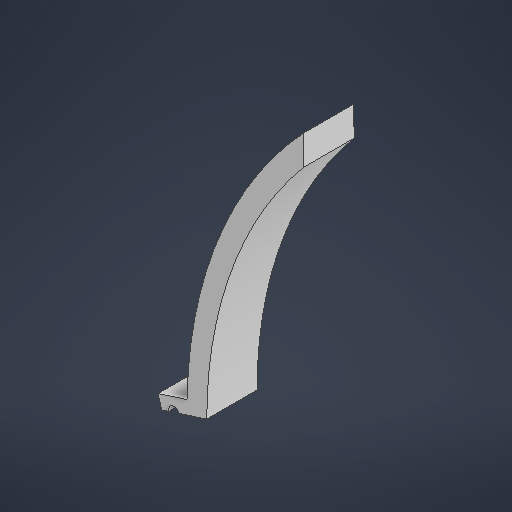
# Autodesk Inventor part: направление
Saved by Autodesk Inventor 2025 (Build 290162000, 162)
## iProperties
Created: 2025-11-04
Part Number: направление
Material: Типовые
Document SubType Name: Modeling
Designer: GameHD
Density: 1 g/cm^3
Appearance: По умолчанию
Author: GameHD
Autodesk Inventor part; units mm, degrees
ref_plane "YZ Plane" through (0, 0, 0) normal (1, 0, 0) x (0, 1, 0)
ref_plane "XZ Plane" through (0, 0, 0) normal (0, 1, 0) x (-1, 0, 0)
ref_plane "XY Plane" through (0, 0, 0) normal (0, 0, 1) x (1, 0, 0)
sketch "Эскиз1" plane through (0, 0, 0) normal (0, 0, 1) x (1, 0, 0)
  circle A0 centre (0, 0) radius 165
  circle A1 centre (0, 0) radius 172.834
  line L0 (-125, 0) -> (-126.5392, 117.7261)
  line L1 (-132.7592, 119.5177) -> (-197.8467, 76.6552)
  line L2 (-165, 0) -> (-153, 0) construction
  line L3 (-134.7038, 9.8338) -> (-172.765, -2.5204) projected
  line L4 (-165, 0) -> (-172.8154, -2.5368)
  point P0 (-172.834, 0)
  point P1 (-126.3868, 106.0725)
  point P2 (-123, 114.4334)
  point P3 (-172.8149, -2.5694)
  dimension "d0" = 330
  dimension "d1" = 345.668
  dimension "d2" = 40
  constraints: 8 end point, 4 point on circle, 2 coincident, 1 centre point, 1 collinear, 1 horizontal, 1 tangent, 3 other
  measures "d1" diameter of A1
  measures "d2" distance of L2.start L0.start
extrude "Выдавливание1" add sketch "Эскиз1" along normal blind 20 contours L3 L4 A1 L0 A0 picked at (-133.2989, 101.385)
sketch "Эскиз2" plane through (0, 0, 0) normal (0, 0, -1) x (-1, 0, 0)
  arc A0 (172.8154, -2.5368) -> (126.5392, 117.7261) centre (0, 0) ccw projected
  arc A1 (165, 0) -> (126.3868, 106.0725) centre (0, 0) ccw projected
  circle A2 centre (0, 0) radius 168.917
  line L0 (172.8154, -2.5368) -> (165, 0) projected
  circle A3 centre (178.0154, -4.2246) radius 2.1
  line L1 (178.0154, -4.2246) -> (172.8154, -2.5368)
  line L2 (160.1198, 6.946) -> (198.8648, -5.6302)
  line L3 (178.0154, -4.2246) -> (182.8662, -5.7992)
  line L4 (182.8662, -5.7992) -> (187.0032, 6.946)
  point P0 (184.4408, -0.9483)
  point P1 (172.8109, 2.8266)
  point P2 (176.018, -3.5763)
  point P3 (180.0128, -4.873)
  dimension "d8" = 337.834
  dimension "d11" = 4.2
  dimension "d12" = 5.2
  dimension "d13" = 5.1
  dimension "d14" = 5.1
  constraints: 8 end point, 2 centre point, 2 collinear, 1 coincident, 1 parallel, 1 perpendicular
  measures "d8" diameter of A2
  measures "d11" diameter of A3
  measures "d12" horizontal distance of L1.start L0.start
  measures "d13" distance between parallel lines of L1 L2
  measures "d14" distance of L1.start L3.end
extrude "Выдавливание2" add sketch "Эскиз2" against normal up to surface (20 mm away) contours A0 L2 L4 L3 A3 L1
